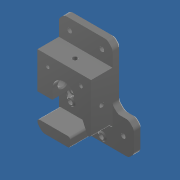
# Autodesk Inventor part: Print_Parts_C
Saved by Autodesk Inventor 2020 (Build 240168000, 168)
## iProperties
Created: 2020-09-26
Part Number: Print_Parts_C
Material: PC/ABS プラスチック
Document SubType Name: Modeling
Designer: rockk
Density: 0.357273 g/cm^3
Appearance: 滑らか - 黒
Author: rockk
Autodesk Inventor part; units mm, degrees
ref_plane "YZ Plane" through (0, 0, 0) normal (1, 0, 0) x (0, 1, 0)
ref_plane "XZ Plane" through (0, 0, 0) normal (0, 1, 0) x (-1, 0, 0)
ref_plane "XY Plane" through (0, 0, 0) normal (0, 0, 1) x (1, 0, 0)
sketch "スケッチ1" plane through (0, 0, 0) normal (0, 0, 1) x (1, 0, 0)
  line L0 (0, 0) -> (-50, 0)
  line L1 (-50, 0) -> (-50, -65)
  line L2 (-50, -65) -> (0, -65)
  line L3 (0, -65) -> (0, 0)
  circle A0 centre (-9.5, -60) radius 1.65
  circle A1 centre (-9.5, -60) radius 6 construction
  circle A2 centre (-9.5, -60) radius 8 construction
  line L4 (-15.5, -60) -> (-17, -60) construction
  line L5 (-23.0862, -25) -> (-21.5862, -25) construction
  circle A3 centre (-25, -25) radius 6 construction
  circle A4 centre (-25, -25) radius 8 construction
  circle A5 centre (-25, -25) radius 11.15
  line L6 (-9.5, -40.5) -> (-40.5, -40.5) construction
  line L7 (-40.5, -40.5) -> (-40.5, -9.5) construction
  line L8 (-9.5, -9.5) -> (-9.5, -40.5) construction
  line L9 (-9.5, -40.5) -> (-40.5, -9.5) construction
  line L10 (-40.5, -40.5) -> (-9.5, -9.5) construction
  circle A6 centre (-40.5, -40.5) radius 1.65
  circle A7 centre (-40.5, -9.5) radius 1.65
  circle A8 centre (-9.5, -9.5) radius 1.65
  circle A9 centre (-9.5, -40.5) radius 1.65
  line L11 (-2.5, -47.5) -> (-47.5, -47.5) construction
  line L12 (-47.5, -47.5) -> (-47.5, -2.5) construction
  line L13 (-47.5, -2.5) -> (-2.5, -2.5) construction
  line L14 (-2.5, -2.5) -> (-2.5, -47.5) construction
  line L15 (-2.5, -47.5) -> (-47.5, -2.5) construction
  line L16 (-47.5, -47.5) -> (-2.5, -2.5) construction
  circle A10 centre (-38.5, -46.5) radius 1.65
  circle A11 centre (-38.5, -46.5) radius 8 construction
  circle A12 centre (-38.5, -46.5) radius 6 construction
  line L17 (-40.5, -9.5) -> (-9.5, -9.5) construction
  line L18 (-6.5943, -21.3921) -> (-5.9731, -22.7574) construction
  line L19 (-15.6458, -12.3268) -> (-16.267, -10.9614) construction
  line L20 (-30.1153, 1.3681) -> (2.8649, -73.1032) construction
  line L21 (2.8649, -73.1032) -> (4.2364, -72.4958) construction
  line L22 (4.2364, -72.4958) -> (-28.7437, 1.9755) construction
  line L23 (-28.7437, 1.9755) -> (-30.1153, 1.3681) construction
  line L24 (-32.5, 19.1523) -> (-32.5, -77.8639) construction
  line L25 (-32.5, -77.8639) -> (-31, -77.8639) construction
  line L26 (-31, -77.8639) -> (-31, 19.1523) construction
  line L27 (-31, 19.1523) -> (-32.5, 19.1523) construction
  line L28 (-72.2018, -52.5) -> (28.6741, -52.5) construction
  line L29 (28.6741, -52.5) -> (28.6741, -54) construction
  line L30 (28.6741, -54) -> (-72.2018, -54) construction
  line L31 (-72.2018, -54) -> (-72.2018, -52.5) construction
  point P0 (-25, -25)
  dimension "d2" = 12
  dimension "d0" = 3.3
  dimension "d1" = 9.5
  dimension "d3" = 16
  dimension "d5" = 12
  dimension "d7" = 16
  dimension "d9" = 22.3
  dimension "d10" = 31
  dimension "d11" = 31
  dimension "d12" = 65
  dimension "d13" = 50
  dimension "d14" = 3.3
  dimension "d15" = 3.3
  dimension "d16" = 3.3
  dimension "d17" = 3.3
  dimension "d18" = 45
  dimension "d19" = 45
  dimension "d22" = 3.3
  dimension "d23" = 16
  dimension "d25" = 12
  dimension "d32" = 25
  dimension "d33" = 25
  dimension "d34" = 1.5
  dimension "d35" = 60
  dimension "d36" = 1.5
  dimension "d136" = 1.5
  constraints: 64 end point, 12 centre point, 12 parallel, 10 coincident, 7 horizontal, 7 perpendicular, 5 midpoint, 4 tangent, 3 horizontal alignment, 3 other
  measures "d0" diameter of A0
  measures "d1" distance from line of L3 A0.centre
  measures "d3" diameter of A2
  measures "d5" diameter of A3
  measures "d7" diameter of A4
  measures "d9" diameter of A5
  measures "d10" distance of L7.end L8.start
  measures "d11" distance of L6.end L7.end
  measures "d12" distance of L0.end L1.end
  measures "d13" distance of L1.end L2.end
  measures "d14" diameter of A6
  measures "d15" diameter of A7
  measures "d16" diameter of A8
  measures "d17" diameter of A9
  measures "d18" distance of L12.end L13.end
  measures "d19" distance of L11.end L12.end
  measures "d22" diameter of A10
  measures "d23" diameter of A11
  measures "d25" diameter of A12
  measures "d32" distance from line of A3.centre L0
  measures "d33" distance from line of L3 A3.centre
  measures "d34" distance of L20.end L21.end
  measures "d35" distance from line of L0 point (-9.5, -60)
  measures "d36" distance of L24.end L25.end
  measures "d136" distance of L28.end L29.end
extrude "押し出し1" add sketch "スケッチ1" along normal blind 8
sketch "スケッチ2" plane through (0, 0, 8) normal (0, 0, 1) x (1, 0, 0)
  line L0 (0, -65) -> (0, 0) projected
  line L1 (0, 0) -> (-50, 0) projected
  line L2 (-50, 0) -> (-50, -65) projected
  line L3 (-50, -65) -> (0, -65) projected
  line L4 (-70, 20) -> (20, 20)
  line L5 (20, 20) -> (20, -85)
  line L6 (20, -85) -> (-70, -85)
  line L7 (-70, -85) -> (-70, 20)
  line L8 (-50, 0) -> (20, 0)
  line L9 (20, 0) -> (20, 20)
  line L10 (20, 20) -> (-50, 20)
  line L11 (-50, 20) -> (-50, 0)
  line L12 (0, -65) -> (20, -65)
  line L13 (20, -65) -> (20, 20)
  line L14 (20, 20) -> (0, 20)
  line L15 (0, 20) -> (0, -65)
  point P0 (20, -65)
  dimension "d37" = 20
  constraints: 24 end point, 4 parallel, 2 horizontal, 2 perpendicular, 3 other
  measures "d37" distance between parallel lines of L1 L4
extrude "押し出し2" add sketch "スケッチ2" against normal up to surface (8 mm away) contours L0 L8 L5 L12 | L15 L4 L5 L8 | L1 L11 L4 L15
sketch "スケッチ3" plane through (0, 0, 8) normal (0, 0, 1) x (1, 0, 0)
  line L0 (-50, 20) -> (-50, -65) projected
  line L1 (-50, -65) -> (20, -65) projected
  line L2 (20, -65) -> (20, 20) projected
  circle A0 centre (-9.5, -60) radius 1.65 projected
  circle A1 centre (-25, -25) radius 11.15 projected
  circle A2 centre (-40.5, -9.5) radius 1.65 projected
  circle A3 centre (-9.5, -9.5) radius 1.65 projected
  circle A4 centre (-38.5, -46.5) radius 1.65 projected
  line L3 (-50, 20) -> (20, 20)
  line L4 (20, 20) -> (20, 0)
  line L5 (20, 0) -> (-50, 0)
  line L6 (-50, 0) -> (-50, 20)
  line L7 (0, -65) -> (20, -65)
  line L8 (20, -65) -> (20, 20)
  line L9 (20, 20) -> (0, 20)
  line L10 (0, 20) -> (0, -65)
  circle A5 centre (-9.5, -60) radius 6
  circle A6 centre (-38.5, -46.5) radius 1.65 projected
  circle A7 centre (-38.5, -46.5) radius 6
  circle A8 centre (-25, -25) radius 6
  line L11 (-44.0665, 32.8709) -> (8.3733, -85.5415)
  line L12 (8.3733, -85.5415) -> (9.7448, -84.9341)
  line L13 (9.7448, -84.9341) -> (-42.695, 33.4783)
  line L14 (-42.695, 33.4783) -> (-44.0665, 32.8709)
  line L15 (-32.5, -46.5) -> (-32.5, -25)
  line L16 (-32.5, -25) -> (-31, -25)
  line L17 (-31, -25) -> (-31, -46.5)
  line L18 (-31, -46.5) -> (-32.5, -46.5)
  line L19 (-37.2043, 30.094) -> (7.2487, -70.2837)
  circle A9 centre (-25, -25) radius 8
  circle A10 centre (-9.5, -60) radius 8
  circle A11 centre (-38.5, -46.5) radius 8
  line L20 (-36.15, -25) -> (-62.2919, -25)
  line L21 (-62.2919, -25) -> (-62.2919, -34)
  line L22 (-62.2919, -34) -> (-36.15, -34)
  line L23 (-36.15, -34) -> (-36.15, -25)
  line L24 (0, 0) -> (0, -65)
  point P0 (-31.75, -46.5)
  point P1 (0, -53.9157)
  point P2 (0, 0)
  point P3 (-50, -34)
  point P4 (-14.805, -20.4851)
  dimension "d40" = 20
  dimension "d41" = 12
  dimension "d42" = 12
  dimension "d43" = 12
  dimension "d44" = 1.5
  dimension "d45" = 1.5
  dimension "d46" = 16
  dimension "d47" = 16
  dimension "d48" = 16
  dimension "d137" = 54
  constraints: 44 end point, 11 parallel, 6 centre point, 6 coincident, 5 perpendicular, 4 tangent, 3 horizontal, 3 horizontal alignment, 2 point on line, 1 collinear, 1 midpoint, 3 other
  measures "d40" distance of L3.end L4.end
  measures "d41" diameter of A5
  measures "d42" diameter of A7
  measures "d43" diameter of A8
  measures "d44" distance of L17.end L15.start
  measures "d45" distance of L11.end L12.end
  measures "d46" diameter of A9
  measures "d47" diameter of A10
  measures "d48" diameter of A11
  measures "d137" distance between parallel lines of L22 L3
extrude "押し出し3" add sketch "スケッチ3" along normal blind 20 contours L5 L11 A1 L20 L0 | L20 L23 L22 L0 | L5 L13 A1 L11 | L5 L19 A1 L13 | L5 L10 L19
sketch "スケッチ4" plane through (0, 0, 8) normal (0, 0, 1) x (1, 0, 0)
  circle A0 centre (-9.5, -40.5) radius 1.65 projected
  circle A1 centre (-40.5, -40.5) radius 1.65 projected
  circle A2 centre (-38.5, -46.5) radius 1.65 projected
  circle A3 centre (-9.5, -40.5) radius 1.65 projected
  circle A4 centre (-40.5, -40.5) radius 1.65 projected
  circle A5 centre (-9.5, -60) radius 1.65 projected
  line L0 (-36.15, -25) -> (-36.15, -34) projected
  line L1 (-36.15, -34) -> (-50, -34) projected
  line L2 (-50, -34) -> (-50, -65) projected
  line L3 (-50, -65) -> (20, -65) projected
  line L4 (20, -65) -> (20, 20) projected
  line L5 (20, 20) -> (-50, 20) projected
  line L6 (-50, 20) -> (-50, 0) projected
  line L7 (-50, 0) -> (0, 0) projected
  line L8 (0, 0) -> (0, -53.9157) projected
  line L9 (0, -53.9157) -> (-14.805, -20.4851) projected
  arc A6 (-36.15, -25) -> (-14.805, -20.4851) centre (-25, -25) ccw projected
hole "穴1" at (-40.5, -40.5, 8) at (-9.5, -40.5, 8) direction (0, 0, -1) diameter 6.5 depth 3
sketch "スケッチ5" plane through (0, 0, 8) normal (0, 0, 1) x (1, 0, 0)
  circle A0 centre (-38.5, -46.5) radius 1.65 projected
  circle A1 centre (-9.5, -60) radius 1.65 projected
  circle A2 centre (-38.5, -46.5) radius 3
  circle A3 centre (-9.5, -60) radius 3
  dimension "d58" = 6
  dimension "d59" = 6
  constraints: 2 centre point, 2 coincident
  measures "d58" diameter of A2
  measures "d59" diameter of A3
extrude "押し出し4" add sketch "スケッチ5" along normal blind 1
chamfer "面取り1" distance 1 angle 45 2 edges at (-41.5, -46.5, 8) (-12.5, -60, 8)
sketch "スケッチ6" plane through (-50, -34, 8) normal (0, -1, 0) x (1, 0, 0)
  line L0 (35.195, 0) -> (13.85, 0) projected
  line L1 (35.195, 0) -> (35.195, 20) projected
  line L2 (13.85, 20) -> (35.195, 20) projected
  line L3 (13.85, 0) -> (13.85, 20) projected
  line L4 (13.85, -8) -> (36.15, -8) projected
  line L5 (8.6947, 0) -> (12.0334, 0) projected
  line L6 (8.6947, 0) -> (12.0334, 0) projected
  line L7 (37.25, 0) -> (43.75, 0) projected
  line L8 (13.85, 0) -> (0, 0) projected
  line L9 (0, 0) -> (70, 0) projected
  line L10 (70, 0) -> (0, 0) projected
  line L11 (0, 0) -> (50, 0) projected
  line L12 (50, 0) -> (35.195, 0) projected
  line L13 (35.195, 0) -> (13.85, 0) projected
  line L14 (44.5, 0) -> (36.5, 0) projected
  line L15 (13.85, 0) -> (36.5, 0) projected
  line L16 (50, 20) -> (0, 20) projected
  line L17 (0, 20) -> (13.85, 20) projected
  line L18 (13.85, 20) -> (35.195, 20) projected
  line L19 (35.195, 20) -> (50, 20) projected
  line L20 (7.85, 20) -> (11.15, 20) projected
  line L21 (38.85, 20) -> (42.15, 20) projected
  line L22 (13.85, -8) -> (36.15, -8) projected
  line L23 (50, 0) -> (50, 20) projected
  point P0 (50, -8)
  point P1 (25, 10)
  point P2 (15.5, 0)
  point P3 (7.5, 0)
  point P4 (6.5, 0)
  point P5 (12.5, 0)
  point P6 (37, 0)
  point P7 (44, 0)
  dimension "d65" = 10
  dimension "d66" = 25
  measures "d65" distance from line of point (25, 10) L2
  measures "d66" distance from line of point (25, 10) L23
hole "穴2" at (-25, -34, 18) direction (0, 1, 0) diameter 4.3 depth 58 counterbore diameter 8 counterbore depth 29
sketch "スケッチ7" plane through (-50, -65, 0) normal (-1, 0, 0) x (0, 0, 1)
  line L0 (28, 65) -> (28, 31) projected
  line L1 (8, 65) -> (28, 65) projected
  line L2 (28, 51.15) -> (0, 51.15) projected
  line L3 (8, 44.5149) -> (28, 44.5149) projected
  line L4 (0, 0) -> (0, 85) projected
  line L5 (0, 0) -> (8, 0) projected
  line L6 (8, 31) -> (8, 0) projected
  line L7 (8, 31) -> (28, 31) projected
  line L8 (28, 65) -> (28, 31) projected
  line L9 (8, 65) -> (28, 65) projected
  line L10 (8, 85) -> (8, 65) projected
  line L11 (8, 85) -> (0, 85) projected
  point P0 (0, 65)
  point P1 (18, 40)
  dimension "d77" = 10
  dimension "d78" = 25
  measures "d77" distance from line of point (18, 40) L0
  measures "d78" distance from line of point (18, 40) L1
hole "穴3" at (-50, -25, 18) direction (1, 0, 0) diameter 4.3 depth 58 counterbore diameter 8 counterbore depth 45
fillet "フィレット2" radius 2 1 edges at (0, -53.9157, 18)
sketch "スケッチ8" plane through (0, 0, 0) normal (0, 0, -1) x (-1, 0, 0)
  line L0 (50, 20) -> (-20, 20) projected
  line L1 (-20, 20) -> (-20, -65) projected
  line L2 (50, -34) -> (50, -65) projected
  line L3 (0, 0) -> (0, -44.4604) projected
  line L4 (50, -65) -> (0, -65)
  line L5 (0, -65) -> (0, 0)
  line L6 (0, 0) -> (50, 0)
  line L7 (50, 0) -> (50, -65)
  line L8 (-20, 20) -> (0, 20)
  line L9 (0, 20) -> (0, -35)
  line L10 (0, -35) -> (-20, -35)
  line L11 (-20, -35) -> (-20, 20)
  point P0 (-20, -35)
  point P1 (0, -35)
  dimension "d88" = 35
  constraints: 16 end point, 4 parallel, 2 horizontal, 2 perpendicular, 1 point on line
  measures "d88" distance between parallel lines of L6 L10
extrude "押し出し5" cut sketch "スケッチ8" against normal blind 10 contours L9 L3 L10 L1 L0
chamfer "面取り3" distance 5 angle 45 6 edges at (20, -65, 4) (20, -35, 4) (-50, 20, 4) (0, -35, 4) (-50, -65, 4) (0, 20, 4)
fillet "フィレット3" radius 5 12 edges at (-50, -60, 4) (-45, -65, 4) (15, -65, 4) (20, -60, 4) (20, -40, 4) (15, -35, 4) (5, -35, 4) (0, -30, 4) (0, 15, 4) (-5, 20, 4) (-45, 20, 4) (-50, 15, 4)
chamfer "面取り4" distance 2 angle 45 24 edges at (-50, -22.5, 0) (-49.6194, 14.8423, 0) (-47.5, 17.5, 0) (-44.8423, 19.6194, 0) (-25, 20, 0) (-5.1577, 19.6194, 0) (-2.5, 17.5, 0) (-0.3806, 14.8423, 0) (0, -7.5, 0) (0.3806, -29.8423, 0) (2.5, -32.5, 0) (5.1577, -34.6194, 0) (10, -35, 0) (14.8423, -35.3806, 0) (17.5, -37.5, 0) (19.6194, -40.1577, 0) (20, -50, 0) (19.6194, -59.8423, 0) (17.5, -62.5, 0) (14.8423, -64.6194, 0) (-15, -65, 0) (-44.8423, -64.6194, 0) (-47.5, -62.5, 0) (-49.6194, -59.8423, 0)
chamfer "面取り7" distance 2 angle 45 6 edges at (-1.5861, -46.4171, 8) (0, -28.9645, 8) (0, -32.5, 8) (0, -39.7302, 8) (-9.3169, -32.8777, 8) (-36.15, -29.5, 8)
sketch "スケッチ9" plane through (0, 0, 28) normal (0, 0, 1) x (1, 0, 0)
  line L0 (0, -44.4604) -> (0, 0) projected
  line L1 (0, -44.4604) -> (2, -44.4604) projected
  arc A0 (-3.8287, -45.2703) -> (0, -44.4604) centre (-2, -44.4604) ccw projected
  arc A1 (-5.6574, -46.0801) -> (2, -44.4604) centre (-2, -44.4604) ccw projected
  arc A2 (0, -27.9289) -> (1.4645, -31.4645) centre (5, -27.9289) ccw projected
  line L2 (0, -27.9289) -> (0, -44.4604) projected
  line L3 (0, -44.4604) -> (2, -44.4604) projected
  line L4 (2, -44.4604) -> (2, -32) projected
  line L5 (1.4645, -31.4645) -> (2, -32) projected
  arc A3 (-3.8287, -45.2703) -> (0, -44.4604) centre (-2, -44.4604) ccw projected
  line L6 (0, -44.4604) -> (0, -65)
  line L7 (-42.9289, -65) -> (12.9289, -65) projected
  line L8 (-3.8287, -45.2703) -> (-5.6574, -46.0801) projected
  point P0 (0, -5)
  point P1 (-3.8287, -44.4059)
  point P2 (0, -47.9245)
  point P3 (2, -44.4604)
  point P4 (0, -27.9289)
  point P5 (0, -47.9245)
  constraints: 2 end point, 1 point on line, 1 vertical, 1 other
extrude "押し出し6" cut sketch "スケッチ9" against normal up to surface (20 mm away) contours L0 A2 L5 L4 L1 | L1 A1 L6
sketch "スケッチ10" plane through (0, 0, 0) normal (0, 0, -1) x (-1, 0, 0)
  line L0 (-20, -42.0711) -> (-20, -57.9289) projected
  line L1 (42.9289, 20) -> (7.0711, 20) projected
  line L2 (0, 12.9289) -> (0, -27.9289) projected
  line L3 (50, -57.9289) -> (50, 12.9289) projected
  line L4 (-20, -57.9289) -> (-20, -42.0711) projected
  point P0 (0, 0)
  point P1 (-10, -50)
  point P2 (10, 10)
  point P3 (40, 10)
  point P4 (-20, -50)
  point P5 (-20, -50)
  dimension "d110" = 10
  dimension "d111" = 10
  dimension "d112" = 10
  dimension "d113" = 10
  constraints: 2 horizontal alignment, 2 midpoint
  measures "d110" distance from line of L0 point (-10, -50)
  measures "d111" distance from line of L1 point (10, 10)
  measures "d112" distance from line of L2 point (10, 10)
  measures "d113" distance from line of point (40, 10) L3
hole "穴4" at (10, -50, 0) at (-10, 10, 0) at (-40, 10, 0) direction (0, 0, 1) diameter 4.3 depth 58 counterbore diameter 8 counterbore depth 4
chamfer "面取り8" distance 1 angle 45 3 edges at (10, -54, 0) (-10, 6, 0) (-40, 6, 0)
sketch "スケッチ11" plane through (0, 0, 8) normal (0, 0, 1) x (1, 0, 0)
  line L0 (-42.9289, -65) -> (12.9289, -65) projected
  arc A0 (-41.3053, -43.6486) -> (-37.9666, -42.5357) centre (-38.5, -46.5) ccw projected
  circle A1 centre (-38.5, -46.5) radius 6
  circle A2 centre (-9.5, -60) radius 1.65 projected
  circle A3 centre (-9.5, -60) radius 6
  line L1 (-66.9185, -52.5) -> (29.4737, -52.5)
  line L2 (29.4737, -52.5) -> (29.4737, -54)
  line L3 (29.4737, -54) -> (-66.9185, -54)
  line L4 (-66.9185, -54) -> (-66.9185, -52.5)
  line L5 (-32.5, -19.3848) -> (-31, -19.3848)
  line L6 (-31, -19.3848) -> (-31, -69.6116)
  line L7 (-31, -69.6116) -> (-32.5, -69.6116)
  line L8 (-32.5, -69.6116) -> (-32.5, -19.3848)
  line L9 (-68.9185, -56) -> (31.4737, -56)
  line L10 (31.4737, -56) -> (31.4737, -50.5)
  line L11 (31.4737, -50.5) -> (-68.9185, -50.5)
  line L12 (-68.9185, -50.5) -> (-68.9185, -56)
  line L13 (-29, -71.6116) -> (-29, -17.3848)
  line L14 (-29, -17.3848) -> (-34.5, -17.3848)
  line L15 (-34.5, -17.3848) -> (-34.5, -71.6116)
  line L16 (-34.5, -71.6116) -> (-29, -71.6116)
  circle A4 centre (-9.5, -60) radius 8
  circle A5 centre (-9.5, -60) radius 10
  line L17 (-19.5, -60) -> (-19.5, -65)
  line L18 (-19.5, -60) -> (-19.5, -56)
  circle A6 centre (10, -50) radius 2.15 projected
  circle A7 centre (-9.5, -60) radius 4 projected
  line L19 (-14.0536, -27.121) -> (-9.5676, -37.2507) projected
  arc A8 (-34.15, -31.3718) -> (-14.0536, -27.121) centre (-25, -25) ccw projected
  arc A9 (-37.9666, -42.5357) -> (-41.3053, -43.6486) centre (-40.5, -40.5) ccw projected
  arc A10 (-41.3053, -43.6486) -> (-37.9666, -42.5357) centre (-38.5, -46.5) ccw projected
  line L20 (-50, -34) -> (-50, -57.9289) projected
  arc A11 (-50, -57.9289) -> (-48.5355, -61.4645) centre (-45, -57.9289) ccw projected
  line L21 (-46.4645, -63.5355) -> (-48.5355, -61.4645) projected
  arc A12 (-46.4645, -63.5355) -> (-42.9289, -65) centre (-42.9289, -60) ccw projected
  line L22 (-42.9289, -65) -> (12.9289, -65) projected
  arc A13 (12.9289, -65) -> (16.4645, -63.5355) centre (12.9289, -60) ccw projected
  line L23 (18.5355, -61.4645) -> (16.4645, -63.5355) projected
  arc A14 (18.5355, -61.4645) -> (20, -57.9289) centre (15, -57.9289) ccw projected
  line L24 (20, -57.9289) -> (20, -42.0711) projected
  arc A15 (20, -42.0711) -> (18.5355, -38.5355) centre (15, -42.0711) ccw projected
  line L25 (16.4645, -36.4645) -> (18.5355, -38.5355) projected
  arc A16 (16.4645, -36.4645) -> (12.9289, -35) centre (12.9289, -40) ccw projected
  line L26 (12.9289, -35) -> (7.0711, -35) projected
  arc A17 (3.5355, -33.5355) -> (7.0711, -35) centre (7.0711, -30) ccw projected
  line L27 (1.4645, -31.4645) -> (3.5355, -33.5355) projected
  line L28 (0, 0) -> (0, 12.9289) projected
  arc A18 (-5.6574, -46.0801) -> (0, -47.9245) centre (-2, -44.4604) ccw projected
  arc A19 (-9.5676, -37.2507) -> (-7.1393, -42.7338) centre (-9.5, -40.5) ccw projected
  arc A20 (-48.5355, 16.4645) -> (-50, 12.9289) centre (-45, 12.9289) ccw projected
  line L29 (-50, 12.9289) -> (-50, 0) projected
  line L30 (-50, 0) -> (0, 0) projected
  arc A21 (0, 12.9289) -> (-1.4645, 16.4645) centre (-5, 12.9289) ccw projected
  line L31 (-3.5355, 18.5355) -> (-1.4645, 16.4645) projected
  arc A22 (-3.5355, 18.5355) -> (-7.0711, 20) centre (-7.0711, 15) ccw projected
  line L32 (-7.0711, 20) -> (-42.9289, 20) projected
  arc A23 (-42.9289, 20) -> (-46.4645, 18.5355) centre (-42.9289, 15) ccw projected
  line L33 (-48.5355, 16.4645) -> (-46.4645, 18.5355) projected
  arc A24 (0, -27.9289) -> (1.4645, -31.4645) centre (5, -27.9289) ccw projected
  line L34 (-34.15, -34) -> (-50, -34) projected
  line L35 (0, -47.9245) -> (0, -27.9289) projected
  line L36 (-7.1393, -42.7338) -> (-5.6574, -46.0801) projected
  line L37 (-34.15, -34) -> (-34.15, -31.3718) projected
  point P0 (0, 0)
  point P1 (-18.1603, -65)
  point P2 (-18.6652, -56)
  point P3 (-29, -56)
  point P4 (-29, -65)
  point P5 (-32.5, -33.2506)
  point P6 (-31, -34.398)
  point P7 (-50, -56)
  dimension "d124" = 12
  dimension "d125" = 12
  dimension "d126" = 1.5
  dimension "d127" = 1.5
  dimension "d128" = 2
  dimension "d129" = 2
  dimension "d130" = 16
  dimension "d131" = 2
  constraints: 36 end point, 8 parallel, 5 perpendicular, 3 centre point, 3 coincident, 3 point on line, 2 horizontal, 2 tangent, 1 vertical, 9 other
  measures "d124" diameter of A1
  measures "d125" diameter of A3
  measures "d126" distance of L1.end L2.end
  measures "d127" distance of L6.end L7.end
  measures "d128" distance between parallel lines of L3 L9
  measures "d129" distance between parallel lines of L6 L13
  measures "d130" diameter of A4
extrude "押し出し7" add sketch "スケッチ11" along normal up to surface (20 mm away) contours A12 L21 A11 L20 L9 L15 L0 | L15 L9 L8 L0 | L8 L9 L6 L0 | L6 L9 L13 L0 | L13 L9 L18 L17 L0
fillet "フィレット7" radius 2 3 edges at (-50, -56, 18) (-19.5, -56, 18) (-19.5, -65, 18)
sketch "スケッチ12" plane through (0, 0, 9) normal (0, 0, 1) x (1, 0, 0)
  circle A0 centre (-38.5, -46.5) radius 3 projected
  circle A1 centre (-9.5, -60) radius 3 projected
  circle A2 centre (-9.5, -60) radius 1.65 projected
  point P0 (-40.128, -43.9802)
  point P1 (-38.7095, -43.5073)
  point P2 (0, 0)
hole "穴5" at (-38.5, -46.5, 9) at (-9.5, -60, 9) direction (0, 0, -1) diameter 4.4 depth 6
sketch "スケッチ13" plane through (-40, 10, 4) normal (0, 0, -1) x (-1, 0, 0)
  circle A0 centre (-30, 0) radius 4 projected
  circle A1 centre (-30, 0) radius 2.15 projected
  circle A2 centre (-50, -60) radius 4 projected
  circle A3 centre (-50, -60) radius 2.15 projected
  circle A4 centre (0, 0) radius 4 projected
  circle A5 centre (0, 0) radius 2.15 projected
  line L0 (-2.15, 2.15) -> (2.15, 2.15)
  line L1 (2.15, 2.15) -> (2.15, -2.15)
  line L2 (2.15, -2.15) -> (-2.15, -2.15)
  line L3 (-2.15, -2.15) -> (-2.15, 2.15)
  line L4 (-2.15, 2.15) -> (2.15, -2.15) construction
  line L5 (2.15, 2.15) -> (-2.15, -2.15) construction
  line L6 (-32.15, 2.15) -> (-27.85, 2.15)
  line L7 (-27.85, 2.15) -> (-27.85, -2.15)
  line L8 (-27.85, -2.15) -> (-32.15, -2.15)
  line L9 (-32.15, -2.15) -> (-32.15, 2.15)
  line L10 (-32.15, 2.15) -> (-27.85, -2.15) construction
  line L11 (-27.85, 2.15) -> (-32.15, -2.15) construction
  line L12 (-52.15, -57.85) -> (-47.85, -57.85)
  line L13 (-47.85, -57.85) -> (-47.85, -62.15)
  line L14 (-47.85, -62.15) -> (-52.15, -62.15)
  line L15 (-52.15, -62.15) -> (-52.15, -57.85)
  line L16 (-52.15, -57.85) -> (-47.85, -62.15) construction
  line L17 (-47.85, -57.85) -> (-52.15, -62.15) construction
  point P0 (-40, -10)
  constraints: 36 end point, 6 midpoint, 6 parallel, 3 horizontal, 3 perpendicular, 1 point on line
extrude "押し出し8" cut sketch "スケッチ13" against normal blind 0.6 contours A1 | L7 L8 A1 | A1 L6 L7 | A1 L9 L6 | L8 L9 A1 | A3 | L13 L14 A3 | A3 L12 L13 | A3 L15 L12 | L14 L15 A3 | A5 | L1 L2 A5 | A5 L0 L1 | A5 L3 L0 | L2 L3 A5
sketch "スケッチ14" plane through (-10, 10, 4) normal (0, 0, -1) x (-1, 0, 0)
  line L0 (-2.15, -2.15) -> (-2.15, 2.15) projected
  line L1 (2.15, 2.15) -> (2.15, -2.15) projected
  circle A0 centre (0, 0) radius 4 projected
  line L2 (27.85, -2.15) -> (27.85, 2.15) projected
  line L3 (27.85, 2.15) -> (32.15, 2.15) projected
  line L4 (32.15, 2.15) -> (32.15, -2.15) projected
  line L5 (32.15, -2.15) -> (27.85, -2.15) projected
  circle A1 centre (30, 0) radius 4 projected
  line L6 (-22.15, -62.15) -> (-22.15, -57.85) projected
  line L7 (-22.15, -57.85) -> (-17.85, -57.85) projected
  line L8 (-17.85, -57.85) -> (-17.85, -62.15) projected
  line L9 (-17.85, -62.15) -> (-22.15, -62.15) projected
  circle A2 centre (-20, -60) radius 4 projected
  line L10 (50.4326, 2.15) -> (-42.605, 2.15)
  line L11 (-42.605, 2.15) -> (-42.605, -2.15)
  line L12 (-42.605, -2.15) -> (50.4326, -2.15)
  line L13 (50.4326, -2.15) -> (50.4326, 2.15)
  line L14 (-12.3346, -57.85) -> (-26.0173, -57.85)
  line L15 (-26.0173, -57.85) -> (-26.0173, -62.15)
  line L16 (-26.0173, -62.15) -> (-12.3346, -62.15)
  line L17 (-12.3346, -62.15) -> (-12.3346, -57.85)
  point P0 (-10, -10)
  point P1 (26.6269, -2.15)
  point P2 (26.6269, 2.15)
  point P3 (33.3731, -2.15)
  point P4 (33.3731, 2.15)
  point P5 (-3.3731, -2.15)
  point P6 (-3.3731, 2.15)
  point P7 (3.3731, -2.15)
  point P8 (3.3731, 2.15)
  point P9 (-16.6269, -62.15)
  point P10 (-16.6269, -57.85)
  point P11 (-23.3731, -62.15)
  point P12 (-23.3731, -57.85)
  constraints: 16 end point, 4 horizontal alignment, 4 parallel, 2 horizontal, 2 perpendicular
extrude "押し出し9" cut sketch "スケッチ14" against normal blind 0.3 contours L12 A0 L10 L0 | L1 L10 A0 L12 | A1 L10 L2 L12 | L12 L4 L10 A1 | L16 A2 L14 L6 | L8 L14 A2 L16
chamfer "面取り9" distance 0.5 angle 45 1 edges at (-50, -25, 14)
chamfer "面取り10" distance 2 angle 45 2 edges at (-12.8055, -25, 14) (-25.0023, -13.85, 22)
sketch "スケッチ16" plane through (-25, -5, 18) normal (0, -1, 0) x (1, 0, 0)
  circle A0 centre (0, 0) radius 4 projected
  circle A1 centre (0, 0) radius 2.15 projected
  point P0 (25, -18)
extrude "押し出し10" cut sketch "スケッチ16" against normal blind 1
sketch "スケッチ17" plane through (-5, -25, 18) normal (-1, 0, 0) x (0, 0, 1)
  circle A0 centre (0, 0) radius 4 projected
  circle A1 centre (0, 0) radius 2.15 projected
  point P0 (-18, 25)
extrude "押し出し11" cut sketch "スケッチ17" against normal blind 1
chamfer "面取り11" distance 1 angle 45 4 edges at (-41.5277, -37.4168, 8) (-8.215, -43.4852, 8) (-12.7498, -40.5338, 8) (-6.5284, -39.184, 9.9961)
sketch "スケッチ18" plane through (0, 0, 0) normal (0, 0, -1) x (-1, 0, 0)
  circle A0 centre (38.5, -46.5) radius 1.65 projected
  circle A1 centre (9.5, -60) radius 1.65 projected
  point P0 (0, 0)
extrude "押し出し12" add sketch "スケッチ18" against normal up to surface (3 mm away)
chamfer "面取り12" distance 1 angle 45 2 edges at (-35.4078, -21, 17.9988) (-36.15, -29, 18)
chamfer "面取り13" distance 1 angle 45 1 edges at (-36.15, -25, 0)
chamfer "面取り15" distance 1 angle 45 4 edges at (-11.15, -40.5, 0) (-11.15, -9.5, 0) (-42.15, -9.5, 0) (-42.15, -40.5, 0)
chamfer "面取り16" distance 1 angle 45 1 edges at (-22.6926, -35.9086, 8)
